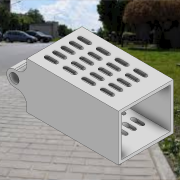
# Autodesk Inventor part: obudowa_WIZ
Saved by Autodesk Inventor 2021 (Build 250183000, 183)
## iProperties
Created: 2025-11-29
Part Number: obudowa_WIZ
Material: Generic
Document SubType Name: Modeling
Designer: huber
Density: 1 g/cm^3
Appearance: Default
Author: huber
Autodesk Inventor part; units mm, degrees
ref_plane "YZ Plane" through (0, 0, 0) normal (1, 0, 0) x (0, 1, 0)
ref_plane "XZ Plane" through (0, 0, 0) normal (0, 1, 0) x (-1, 0, 0)
ref_plane "XY Plane" through (0, 0, 0) normal (0, 0, 1) x (1, 0, 0)
sketch "Sketch1" plane through (0, 0, 0) normal (1, 0, 0) x (0, 1, 0)
  line L0 (22.5, 26.5) -> (-22.5, 26.5)
  line L1 (-22.5, 26.5) -> (-22.5, -26.5)
  line L2 (-22.5, -26.5) -> (22.5, -26.5)
  line L3 (22.5, -26.5) -> (22.5, 26.5)
  line L4 (22.5, 26.5) -> (-22.5, -26.5) construction
  line L5 (-22.5, 26.5) -> (22.5, -26.5) construction
  line L6 (19.5, 23.5) -> (-19.5, 23.5)
  line L7 (-19.5, 23.5) -> (-19.5, -23.5)
  line L8 (-19.5, -23.5) -> (19.5, -23.5)
  line L9 (19.5, -23.5) -> (19.5, 23.5)
  line L10 (19.5, 23.5) -> (-41.0406, -49.4591) construction
  line L11 (-19.5, 23.5) -> (41.0029, -49.4138) construction
  line L12 (-57.4493, 0) -> (57.4117, 0) projected
  line L13 (0, -64.651) -> (0, 41.6918) projected
  line L14 (22.5, -23) -> (23, -23.5)
  point P0 (0, 0)
  point P1 (-8, 23.5)
  point P2 (8, 23.5)
  point P3 (7, -23.5)
  dimension "d0" = 45
  dimension "d1" = 53
  dimension "d2" = 3
  dimension "d48" = 3
  dimension "d49" = 3
  dimension "d50" = 3
  constraints: 26 end point, 6 point on line, 4 parallel, 2 horizontal, 2 midpoint, 2 perpendicular
  measures "d0" distance of L1.end L2.end
  measures "d1" distance of L0.end L1.end
  measures "d2" distance between parallel lines of L2 L8
  measures "d48" distance between parallel lines of L9 L3
  measures "d49" distance between parallel lines of L0 L6
  measures "d50" distance between parallel lines of L1 L7
extrude "Extrusion1" add sketch "Sketch1" along normal blind 85
extrude "Extrusion2" add sketch "Sketch1" against normal blind 3
sketch "Sketch3" plane through (85, -22.5, -26.5) normal (0, -1, 0) x (1, 0, 0)
  line L0 (-88, 53) -> (0, 53) projected
  line L1 (-42.5, 53) -> (-42.5, 0) construction
  line L2 (0, 0) -> (-88, 0) projected
  line L3 (0, 53) -> (0, 0) projected
  point P0 (-85, 26.5)
  dimension "d16" = 42.5
  constraints: 2 end point, 2 point on line, 1 vertical
  measures "d16" distance between parallel lines of L3 L1
ref_plane "Work Plane1" through (42.5, -22.5, 26.5) normal (0.7071068, -0.7071068, 0) x (0, 0, -1)
sketch "Sketch5" plane through (42.5, -22.5, 26.5) normal (0.7071068, -0.7071068, 0) x (0, 0, -1)
  line L0 (0, 0) -> (53, 0) construction
  line L1 (26.5, 0) -> (26.5, 3.2791) construction
  line L2 (26.5, 0) -> (26.5, 13.5441)
  line L3 (26.5, 0) -> (26.5, 5) construction
  line L4 (28.5, 0) -> (28.5, 5)
  line L5 (24.5, 5) -> (24.5, 0)
  arc A0 (24.5, 0) -> (28.5, 0) centre (26.5, 0) ccw
  arc A1 (28.5, 5) -> (24.5, 5) centre (26.5, 5) ccw
  point P0 (26.5, -14.1421)
  point P1 (26.5, 2.5)
  dimension "d19" = 4
  dimension "d20" = 5
  constraints: 12 end point, 4 point on circle, 4 tangent, 2 centre point, 2 midpoint, 2 vertical, 1 parallel, 1 point on line
  measures "d19" distance between parallel lines of L4 L5
  measures "d20" distance of L1.start L3.end
extrude "Extrusion3" cut sketch "Sketch5" along normal blind 33 and the other way blind 7
pattern_linear "Rectangular Pattern1" count 5 spacing 8 along (0, 0, 1) count 4 spacing 18 along (-1, 0, 0) of "Extrusion3" first direction both ways yes second direction both ways yes
mirror "Mirror1" about plane through (0, 0, 0) normal (0, 1, 0) of "Extrusion3", "Rectangular Pattern1"
ref_plane "Work Plane2" through (78.5, 0, 0) normal (1, 0, 0) x (0, 0, -1)
sketch "Sketch12" plane through (85, 0, 0) normal (1, 0, 0) x (0, 0, -1)
  line L0 (23.5, 19.5) -> (-23.5, 19.5)
  line L1 (-23.5, 19.5) -> (-23.5, -19.5)
  line L2 (-23.5, -19.5) -> (23.5, -19.5)
  line L3 (23.5, -19.5) -> (23.5, 19.5)
  line L4 (23.5, 19.5) -> (-23.5, -19.5) construction
  line L5 (-23.5, 19.5) -> (23.5, -19.5) construction
  line L6 (-26.5, -22.5) -> (26.5, -22.5) projected
  line L7 (-26.5, 22.5) -> (-26.5, -22.5) projected
  point P0 (0, 0)
  dimension "d79" = 3
  dimension "d80" = 3
  constraints: 12 end point, 2 midpoint, 2 parallel, 1 horizontal, 1 perpendicular
  measures "d79" distance between parallel lines of L6 L2
  measures "d80" distance between parallel lines of L1 L7
extrude "Extrusion11" cut sketch "Sketch12" against normal blind 86
sketch "Sketch13" plane through (85, -22.5, 26.5) normal (0, 0, 1) x (1, 0, 0)
  line L0 (-88, 0) -> (0, 0) projected
  line L1 (0, 45) -> (0, 0) projected
  line L2 (-88, 45) -> (0, 45) projected
  line L3 (-88, 0) -> (-88, 45) projected
  line L4 (0, 22.5) -> (-88, 22.5)
  circle A0 centre (-100, 22.5) radius 7.5
  line L5 (-100, 22.5) -> (-88, 22.5) construction
  line L6 (-100, 15) -> (-88, 15)
  line L7 (-100, 30) -> (-88, 30)
  line L8 (-88, 0) -> (-88, 45) projected
  point P0 (-85, 22.5)
  dimension "d85" = 15
  dimension "d86" = 12
  constraints: 8 end point, 2 horizontal, 2 midpoint, 2 point on circle, 2 point on line, 2 tangent, 1 centre point, 1 parallel
  measures "d85" diameter of A0
  measures "d86" distance from line of L3 L5.start
extrude "Extrusion12" add sketch "Sketch13" against normal blind 15 contours L6 A0 L7 L3 | A0
sketch "Sketch14" plane through (85, -22.5, 11.5) normal (0, 0, -1) x (-1, 0, 0)
  arc A0 (100, 15) -> (100, 30) centre (100, 22.5) ccw projected
  point P0 (85, 22.5)
  constraints: 1 coincident
hole "Hole2" at (-15, 0, 11.5) direction (0, 0, 1) diameter 9 end through all clearance for "Socket Head Cap Screw ISO 4762" size "M8" standard "ISO"
fillet "Fillet3" radius 10 2 edges at (-3, -7.5, 19) (-3, 7.5, 19)
body "Solid1"
